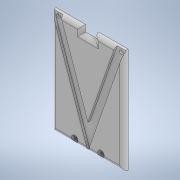
# Autodesk Inventor part: holo - laser battery backing
Saved by Autodesk Inventor 2022 (Build 260153000, 153)
## iProperties
Created: 2022-04-08
Part Number: holo - laser battery backing
Material: Generic
Document SubType Name: Modeling
Designer: chris
Density: 1 g/cm^3
Appearance: Default
Author: chris
Autodesk Inventor part; units mm, degrees
ref_plane "YZ Plane" through (0, 0, 0) normal (1, 0, 0) x (0, 1, 0)
ref_plane "XZ Plane" through (0, 0, 0) normal (0, 1, 0) x (-1, 0, 0)
ref_plane "XY Plane" through (0, 0, 0) normal (0, 0, 1) x (1, 0, 0)
sketch "Sketch1" plane through (0, 0, 0) normal (0, 0, 1) x (1, 0, 0)
  line L0 (-27.94, 0) -> (27.94, 0)
  line L1 (-27.94, 0) -> (-27.94, 76.2)
  line L2 (-27.94, 76.2) -> (-27.94, 81.28)
  line L3 (-27.94, 81.28) -> (27.94, 81.28)
  line L4 (27.94, 81.28) -> (27.94, 0)
  line L5 (-27.94, 76.2) -> (27.94, 76.2)
  line L6 (0, 0) -> (0, 3.5814)
  line L7 (0, 3.5814) -> (-10.16, 3.5814)
  line L8 (-10.16, 3.5814) -> (10.16, 3.5814)
  circle A0 centre (-10.16, 3.5814) radius 1.524
  circle A1 centre (10.16, 3.5814) radius 1.524
  line L9 (0, 76.2) -> (0, 81.28)
  line L10 (0, 76.2) -> (-5.08, 76.2)
  line L11 (-5.08, 76.2) -> (-5.08, 81.28)
  line L12 (0, 76.2) -> (5.08, 76.2)
  line L13 (5.08, 76.2) -> (5.08, 81.28)
  dimension "d0" = 55.88
  dimension "d1" = 76.2
  dimension "d2" = 5.08
  dimension "d3" = 3.5814
  dimension "d4" = 10.16
  dimension "d5" = 20.32
  dimension "d6" = 3.048
  dimension "d7" = 3.048
  dimension "d8" = 5.08
  constraints: 28 end point, 7 point on line, 5 perpendicular, 3 coincident, 3 midpoint, 2 centre point, 2 horizontal, 2 vertical
  measures "d0" distance of L0.start L0.end
  measures "d1" distance of L0.start L1.end
  measures "d2" distance of L1.end L2.end
  measures "d3" distance of L6.start L6.end
  measures "d4" distance of L6.end L7.end
  measures "d5" distance of L7.end L8.end
  measures "d6" diameter of A0
  measures "d7" diameter of A1
  measures "d8" distance of L9.start L12.end
extrude "Extrusion1" add sketch "Sketch1" along normal blind 3.175 contours L1 L5 L4 L0 | L2 L3 L11 L5 | L5 L13 L3 L4
sketch "Sketch2" plane through (0, 0, 3.175) normal (0, 0, 1) x (1, 0, 0)
  line L0 (-27.94, 81.28) -> (-27.94, 0) projected
  line L1 (3.4628, 9.8032) -> (-34.29, 119.2864)
  line L2 (-34.29, 119.2864) -> (-34.29, 0)
  line L3 (0, 0) -> (0, 76.2)
  line L4 (5.08, 76.2) -> (-5.08, 76.2) projected
  line L5 (-3.4628, 9.8032) -> (34.29, 119.2864)
  line L6 (27.94, 0) -> (27.94, 81.28) projected
  line L7 (27.94, 81.28) -> (5.08, 81.28) projected
  line L8 (5.08, 81.28) -> (5.08, 76.2) projected
  line L9 (5.08, 76.2) -> (-5.08, 76.2) projected
  line L10 (-5.08, 76.2) -> (-5.08, 81.28) projected
  line L11 (-5.08, 81.28) -> (-27.94, 81.28) projected
  line L12 (-27.94, 81.28) -> (-27.94, 0) projected
  line L13 (-27.94, 0) -> (27.94, 0) projected
  circle A0 centre (-10.16, 3.5814) radius 1.524 projected
  circle A1 centre (10.16, 3.5814) radius 1.524 projected
  line L14 (0, 0) -> (0, 0.254)
  line L15 (-5.08, 81.28) -> (-27.94, 81.28) projected
  line L16 (0, 0.254) -> (-27.94, 81.28)
  line L17 (0, 0.254) -> (27.94, 81.28)
  point P0 (6.0051, 2.0643)
  point P1 (-6.0051, 2.0643)
  point P2 (21.1843, 81.28)
  point P3 (0, 19.8454)
  point P4 (-21.1843, 81.28)
  dimension "d15" = 0.254
  constraints: 14 end point, 3 symmetric about line, 2 parallel, 1 midpoint, 1 point on line
  measures "d15" distance of L3.start L14.end
extrude "Extrusion2" cut sketch "Sketch2" against normal blind 1.5875 contours L11 L1 L5 L16 | L5 L3 L16 | L5 L7 L17 L1 | L1 L17 L3 | A0 | A1
fillet "Fillet1" radius 3.175 8 edges at (-13.1322, 81.28, 3.175) (13.1322, 81.28, 3.175) (27.94, 40.64, 3.175) (-27.94, 40.64, 3.175) (-5.08, 78.74, 3.175) (0, 76.2, 3.175) (5.08, 78.74, 3.175) (0, 0, 3.175)
sketch "Sketch3" plane through (0, 0, 1.5875) normal (0, 0, 1) x (1, 0, 0)
  line L0 (0.0591, 0.4254) -> (-0.0591, 0.4254) projected
  line L1 (27.5146, 80.0464) -> (0.0591, 0.4254) projected
  line L2 (27.5146, 80.8546) -> (27.5146, 80.0464) projected
  line L3 (21.0377, 80.8546) -> (27.5146, 80.8546) projected
  line L4 (0, 19.8454) -> (21.0377, 80.8546) projected
  line L5 (-21.0377, 80.8546) -> (0, 19.8454) projected
  line L6 (-27.5146, 80.8546) -> (-21.0377, 80.8546) projected
  line L7 (-27.5146, 80.0464) -> (-27.5146, 80.8546) projected
  line L8 (-0.0591, 0.4254) -> (-27.5146, 80.0464) projected
  circle A0 centre (-24.2761, 78.105) radius 1.524
  line L9 (-27.5146, 80.8546) -> (-27.94, 81.28) projected
  line L10 (-27.5146, 80.8546) -> (-21.0377, 80.8546) projected
  line L11 (-21.0377, 80.8546) -> (-20.0895, 78.105) projected
  line L12 (-20.0895, 78.105) -> (-8.255, 78.105) projected
  line L13 (-8.255, 78.105) -> (-5.08, 81.28) projected
  line L14 (-5.08, 81.28) -> (-27.94, 81.28) projected
  line L15 (-27.94, 81.28) -> (-27.94, 0) projected
  line L16 (5.08, 76.2) -> (-5.08, 76.2) projected
  line L17 (0, 76.2) -> (0, 83.5529)
  circle A1 centre (24.2761, 78.105) radius 1.524
  line L18 (-1.0072, 3.175) -> (-8.6912, 3.175) projected
  line L19 (-1.0072, 3.175) -> (-24.765, 72.0725) projected
  line L20 (-24.765, 3.175) -> (-24.765, 72.0725) projected
  line L21 (-11.6288, 3.175) -> (-24.765, 3.175) projected
  arc A2 (-8.6912, 3.175) -> (-11.6288, 3.175) centre (-10.16, 3.5814) ccw projected
  line L22 (8.6912, 3.175) -> (1.0072, 3.175) projected
  arc A3 (11.6288, 3.175) -> (8.6912, 3.175) centre (10.16, 3.5814) ccw projected
  line L23 (24.765, 3.175) -> (11.6288, 3.175) projected
  line L24 (24.765, 72.0725) -> (24.765, 3.175) projected
  line L25 (24.765, 72.0725) -> (1.0072, 3.175) projected
  point P0 (0, 0)
  point P1 (-24.2761, 80.8546)
  dimension "d16" = 3.048
  dimension "d17" = 3.175
  dimension "d21" = 74.5236
  dimension "d22" = 14.1161
  constraints: 2 centre point, 2 end point, 2 midpoint, 1 symmetric about line, 1 vertical, 1 vertical alignment, 1 other
  measures "d16" diameter of A0
  measures "d17" distance from line of L14 A0.centre
  measures "d21" vertical distance of A2.centre A0.centre
  measures "d22" horizontal distance of A2.centre A0.centre
extrude "Extrusion3" cut sketch "Sketch3" against normal blind 25.4 contours A0 | A1
sketch "Sketch4" plane through (0, 0, 3.175) normal (0, 0, 1) x (1, 0, 0)
  line L0 (-1.0072, 3.175) -> (-8.6912, 3.175) projected
  line L1 (-1.0072, 3.175) -> (-24.765, 72.0725) projected
  line L2 (-24.765, 3.175) -> (-24.765, 72.0725) projected
  line L3 (-11.6288, 3.175) -> (-24.765, 3.175) projected
  arc A0 (-8.6912, 3.175) -> (-11.6288, 3.175) centre (-10.16, 3.5814) ccw projected
  line L4 (8.6912, 3.175) -> (1.0072, 3.175) projected
  arc A1 (11.6288, 3.175) -> (8.6912, 3.175) centre (10.16, 3.5814) ccw projected
  line L5 (24.765, 3.175) -> (11.6288, 3.175) projected
  line L6 (24.765, 72.0725) -> (24.765, 3.175) projected
  line L7 (24.765, 72.0725) -> (1.0072, 3.175) projected
  circle A2 centre (-10.16, 3.5814) radius 1.524 projected
  circle A3 centre (-10.16, 3.5814) radius 2.5
  arc A4 (11.6288, 3.175) -> (8.6912, 3.175) centre (10.16, 3.5814) ccw projected
  circle A5 centre (10.16, 3.5814) radius 2.5
  point P0 (0, 0)
  point P1 (12.6267, 3.175)
  point P2 (7.6933, 3.175)
  dimension "d23" = 5
  dimension "d24" = 5
  constraints: 2 centre point, 2 coincident
  measures "d23" diameter of A3
  measures "d24" diameter of A5
extrude "Extrusion4" cut sketch "Sketch4" against normal blind 1.5875 contours A3 L3 A2 L0 | L0 A0 L3 A3 | A2 A0 | A1 L5 A5 L4 | L4 A5 L5 A1
body "Solid1"
